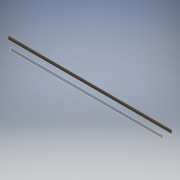
# Autodesk Inventor part: Brett_vorne
Saved by Autodesk Inventor 2017 (Build 210142000, 142)
## iProperties
Created: 2017-05-11
Part Number: Brett_vorne
Material: Generic
Document SubType Name: Modeling
Designer: Fake
Density: 1 g/cm^3
Appearance: Treibholz
Author: Fake
Autodesk Inventor part; units mm, degrees
ref_plane "YZ Plane" through (0, 0, 0) normal (1, 0, 0) x (0, 1, 0)
ref_plane "XZ Plane" through (0, 0, 0) normal (0, 1, 0) x (-1, 0, 0)
ref_plane "XY Plane" through (0, 0, 0) normal (0, 0, 1) x (1, 0, 0)
ref_plane "Arbeitsebene1" through (-659.8695, -810.8277, 426.2571) normal (0, 1, 0) x (-1, 0, 0)
sketch "Skizze1" plane through (-659.8695, -810.8277, 426.2571) normal (0, 1, 0) x (-1, 0, 0)
  line L0 (323.9176, 363.1286) -> (-4356.0824, 363.1286)
  line L1 (-4356.0824, 363.1286) -> (-4356.0824, 263.1286)
  line L2 (-4356.0824, 263.1286) -> (323.9176, 263.1286)
  line L3 (323.9176, 263.1286) -> (323.9176, 363.1286)
  dimension "d0" = 4680
  dimension "d1" = 100
  constraints: 8 end point, 2 parallel, 1 horizontal, 1 perpendicular
  measures "d0" distance of L0.start L0.end
  measures "d1" distance of L2.end L0.start
extrude "Extrusion1" add sketch "Skizze1" against normal blind 15
sketch "Skizze2" plane through (3696.2129, -810.8277, 789.3857) normal (1, 0, 0) x (0, 0, -1)
  line L0 (0, 0) -> (100, 0) projected
  line L1 (0, 0) -> (0, -15) projected
  line L2 (100, -15) -> (0, -15) projected
  line L3 (100, 0) -> (100, -15) projected
  line L4 (0, -15) -> (100, -15) projected
  line L5 (0, -15) -> (11, -15)
  line L6 (11, -15) -> (11, -9)
  line L7 (11, -9) -> (0, -9)
  line L8 (0, -9) -> (0, -15)
  line L9 (100, 0) -> (0, 0) projected
  line L10 (11, 0) -> (0, 0)
  line L11 (0, 0) -> (0, -4)
  line L12 (0, -4) -> (11, -4)
  line L13 (11, -4) -> (11, 0)
  line L14 (100, 0) -> (100, -15) projected
  line L15 (100, -7.5) -> (90, -7.5)
  line L16 (90, -7.5) -> (90, -4)
  line L17 (90, -4) -> (100, -4)
  line L18 (100, -4) -> (100, -7.5)
  line L19 (0, -15) -> (100, -15)
  line L20 (100, -15) -> (100, 0)
  line L21 (100, 0) -> (0, 0)
  line L22 (0, 0) -> (0, -15)
  dimension "d4" = 5
  dimension "d5" = 11
  dimension "d6" = 4
  dimension "d7" = 10
  constraints: 32 end point, 8 parallel, 4 horizontal, 4 perpendicular, 4 point on line, 1 midpoint
  measures "d4" distance between parallel lines of L12 L7
  measures "d5" distance of L6.end L7.end
  measures "d6" distance between parallel lines of L0 L12
  measures "d7" distance between parallel lines of L3 L16
extrude "Extrusion2" cut sketch "Skizze2" against normal up to surface (4680 mm away) contours L0 L13 L12 L1 | L7 L6 L2 L1 | L3 L15 L16 L17
chamfer "Fase1" distance 2 angle 45 1 edges at (1356.2129, -825.8277, 778.3857)
chamfer "Fase2" distance 1 angle 45 3 edges at (1356.2129, -814.8277, 789.3857) (1356.2129, -819.8277, 789.3857) (1356.2129, -810.8277, 778.3857)
